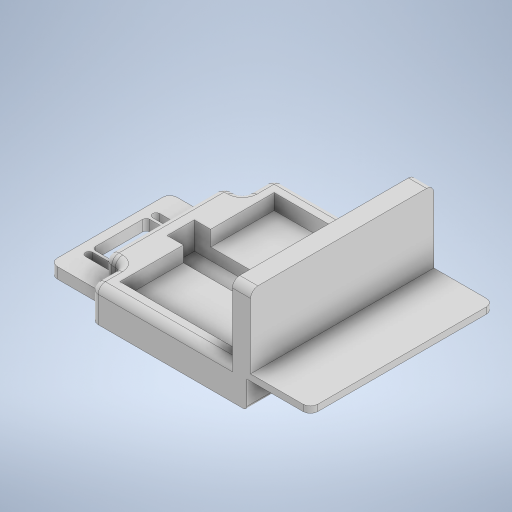
# Autodesk Inventor part: frame
Saved by Autodesk Inventor 2024 (Build 280153000, 153)
## iProperties
Created: 2024-11-23
Part Number: frame
Material: Generic
Document SubType Name: Modeling
Designer: tibs0
Density: 1 g/cm^3
Appearance: Default
Author: tibs0
Autodesk Inventor part; units mm, degrees
ref_plane "YZ Plane" through (0, 0, 0) normal (1, 0, 0) x (0, 1, 0)
ref_plane "XZ Plane" through (0, 0, 0) normal (0, 1, 0) x (-1, 0, 0)
ref_plane "XY Plane" through (0, 0, 0) normal (0, 0, 1) x (1, 0, 0)
sketch "Sketch1" plane through (0, 0, 0) normal (0, 1, 0) x (-1, 0, 0)
  line L0 (-35, 42.5) -> (35, 42.5)
  line L1 (35, 42.5) -> (35, -42.5)
  line L2 (35, -42.5) -> (-35, -42.5)
  line L3 (-35, -42.5) -> (-35, 42.5)
  line L4 (-35, 42.5) -> (35, -42.5) construction
  line L5 (35, 42.5) -> (-35, -42.5) construction
  line L6 (43, -50.5) -> (43, 50.5)
  line L7 (43, 50.5) -> (-43, 50.5)
  line L8 (-43, 50.5) -> (-43, -50.5)
  line L9 (-43, -50.5) -> (43, -50.5)
  line L10 (-43, -50.5) -> (-78, -50.5)
  line L11 (-78, -50.5) -> (-78, 50.5)
  line L12 (-78, 50.5) -> (-43, 50.5)
  line L13 (-43, 50.5) -> (-43, -50.5)
  point P0 (0, 0)
  point P1 (-43, 50.5)
  dimension "d0" = 70
  dimension "d1" = 85
  dimension "d2" = 8
  dimension "d13" = 35
  constraints: 28 end point, 6 parallel, 3 perpendicular, 2 horizontal, 2 midpoint, 3 other
  measures "d0" distance of L1.end L2.end
  measures "d1" distance of L0.end L1.end
  measures "d2" distance between parallel lines of L1 L6
  measures "d13" distance of L11.end L12.end
extrude "Extrusion1" add sketch "Sketch1" along normal blind 10 contours L0 L1 L2 L3
extrude "Extrusion2" add sketch "Sketch1" along normal blind 18.5
sketch "Sketch5" plane through (-43, 0, 50.5) normal (0, 0, 1) x (1, 0, 0)
  line L0 (0, 0) -> (121, 0) projected
  line L1 (121, 0) -> (121, 18.5) projected
  line L2 (0, 18.5) -> (121, 18.5) projected
  line L3 (0, 0) -> (0, 18.5) projected
  line L4 (78, 10) -> (78, 18.5) projected
  line L5 (121, 0) -> (86, 0)
  line L6 (86, 0) -> (86, 15)
  line L7 (86, 15) -> (121, 15)
  line L8 (121, 15) -> (121, 0)
  point P0 (43, 0)
  point P1 (86, 0)
  dimension "d14" = 35
  dimension "d15" = 15
  constraints: 8 end point, 2 parallel, 1 horizontal, 1 perpendicular
  measures "d14" distance of L6.end L7.end
  measures "d15" distance of L5.end L6.end
extrude "Extrusion5" cut sketch "Sketch5" against normal blind 101 contours L6 L7 L1 L0
sketch "Sketch6" plane through (0, 18.5, 0) normal (0, 1, 0) x (1, 0, 0)
  line L0 (-43, -50.5) -> (78, -50.5) projected
  line L1 (78, -50.5) -> (78, 50.5) projected
  line L2 (78, 50.5) -> (-43, 50.5) projected
  line L3 (-43, 50.5) -> (-43, -50.5) projected
  line L4 (35, -42.5) -> (-35, -42.5) projected
  line L5 (-35, -42.5) -> (-35, 42.5) projected
  line L6 (-35, 42.5) -> (35, 42.5) projected
  line L7 (35, 42.5) -> (35, -42.5) projected
  line L8 (35, 50.5) -> (45, 50.5)
  line L9 (45, 50.5) -> (45, -50.5)
  line L10 (45, -50.5) -> (35, -50.5)
  line L11 (35, -50.5) -> (35, 50.5)
  point P0 (0, 0)
  point P1 (35, -42.5)
  dimension "d18" = 10
  dimension "d21" = 0
  constraints: 8 end point, 2 parallel, 2 point on line, 1 horizontal, 1 perpendicular
  measures "d18" distance of L9.end L10.end
  measures "d21" distance between parallel lines of L7 L11
extrude "Extrusion6" add sketch "Sketch6" along normal blind 40 contours L11 L7 L2 L9 L0
sketch "Sketch8" plane through (-43, 18.5, 50.5) normal (0, 0, 1) x (1, 0, 0)
  line L0 (86, -3.5) -> (121, -3.5) projected
  line L1 (121, -3.5) -> (121, 0) projected
  line L2 (88, 0) -> (121, 0) projected
  line L3 (88, 0) -> (88, 40) projected
  line L4 (78, 40) -> (88, 40) projected
  line L5 (78, 0) -> (78, 40) projected
  line L6 (0, 0) -> (78, 0) projected
  line L7 (0, -18.5) -> (0, 0) projected
  line L8 (0, -18.5) -> (86, -18.5) projected
  line L9 (86, -18.5) -> (86, -3.5) projected
  line L10 (121, -3.5) -> (86, -3.5) projected
  line L11 (101.2519, -3.5) -> (101.2519, -33.5)
  line L12 (101.2519, -33.5) -> (-48.597, -33.5)
  line L13 (-48.597, -30.5) -> (-20.6061, -30.5)
  line L14 (-48.597, -27.5) -> (-20.6061, -27.5)
  point P0 (43, -18.5)
  dimension "d25" = 30
  dimension "d26" = 3
  dimension "d27" = 3
  constraints: 8 end point, 2 perpendicular, 1 horizontal, 1 parallel, 1 point on line
  measures "d25" distance of L11.start L11.end
  measures "d26" distance between parallel lines of L12 L13
  measures "d27" distance between parallel lines of L13 L14
sketch "Sketch9" plane through (-43, 0, -50.5) normal (-1, 0, 0) x (0, 0, 1)
  line L0 (0, 0) -> (101, 0) projected
  line L1 (101, 0) -> (101, 18.5) projected
  line L2 (0, 18.5) -> (101, 18.5) projected
  line L3 (0, 0) -> (0, 18.5) projected
  point P0 (50.5, 0)
extrude "Extrusion8" add sketch "Sketch9" along normal blind 40
sketch "Sketch10" plane through (0, 0, 0) normal (0, -1, 0) x (1, 0, 0)
  line L0 (43, -50.5) -> (43, 50.5) projected
  line L1 (-83, 50.5) -> (43, 50.5) projected
  line L2 (-83, -50.5) -> (-83, 50.5) projected
  line L3 (43, -50.5) -> (-83, -50.5) projected
  line L4 (-43, 50.5) -> (-43, -50.5)
  line L5 (43, -50.5) -> (-83, -50.5) projected
  point P0 (0, 0)
  point P1 (-43, -50.5)
  constraints: 2 end point, 1 perpendicular, 1 point on line
extrude "Extrusion9" add sketch "Sketch10" along normal blind 7 contours L3 L2 L1 L4
sketch "Sketch11" plane through (-83, 0, -50.5) normal (-1, 0, 0) x (0, 0, 1)
  line L0 (101, 18.5) -> (101, -7) projected
  line L1 (101, 18.5) -> (0, 18.5) projected
  line L2 (0, 18.5) -> (0, -7) projected
  line L3 (101, -7) -> (0, -7) projected
  line L4 (50.5, -7) -> (83.5, -7)
  line L5 (0, -7) -> (101, -7) projected
  line L6 (50.5, -7) -> (17.5, -7)
  line L7 (17.5, -1) -> (32, -1)
  line L8 (83.5, -1) -> (69, -1)
  line L9 (17.5, -7) -> (17.5, 18.5)
  line L10 (83.5, -7) -> (83.5, 18.5)
  line L11 (32, -1) -> (69, -1)
  line L12 (32, -1) -> (32, -7)
  line L13 (69, -1) -> (69, -7)
  point P0 (50.5, 0)
  dimension "d32" = 33
  dimension "d33" = 33
  dimension "d34" = 14.5
  dimension "d36" = 14.5
  dimension "d39" = 6
  dimension "d40" = 6
  constraints: 18 end point, 6 point on line, 4 perpendicular, 2 horizontal, 1 midpoint
  measures "d32" distance of L4.start L4.end
  measures "d33" distance of L4.start L6.end
  measures "d34" distance of L7.start L7.end
  measures "d36" distance of L8.start L8.end
  measures "d39" distance between parallel lines of L3 L7
  measures "d40" distance between parallel lines of L3 L8
extrude "Extrusion10" cut sketch "Sketch11" against normal blind 40 contours L0 L3 L10 L1 | L9 L3 L2 L1
extrude "Extrusion11" cut sketch "Sketch11" against normal blind 30 contours L10 L8 L11 L7 L9 L1
sketch "Sketch12" plane through (-83, -1, 33) normal (0, 1, 0) x (1, 0, 0)
  line L0 (0, 0) -> (0, 66) projected
  line L1 (30, 0) -> (0, 0) projected
  line L2 (30, 0) -> (30, 66) projected
  line L3 (0, 66) -> (30, 66) projected
  line L4 (5, 48) -> (30, 48)
  line L5 (30, 48) -> (30, 18)
  line L6 (30, 18) -> (5, 18)
  line L7 (5, 18) -> (5, 48)
  line L8 (5, 48) -> (30, 18) construction
  line L9 (30, 48) -> (5, 18) construction
  line L10 (5, 53.5) -> (30, 53.5)
  line L11 (30, 53.5) -> (30, 49.5)
  line L12 (30, 49.5) -> (5, 49.5)
  line L13 (5, 49.5) -> (5, 53.5)
  line L14 (5, 53.5) -> (30, 49.5) construction
  line L15 (30, 53.5) -> (5, 49.5) construction
  line L16 (5, 16.5) -> (30, 16.5)
  line L17 (30, 16.5) -> (30, 12.5)
  line L18 (30, 12.5) -> (5, 12.5)
  line L19 (5, 12.5) -> (5, 16.5)
  line L20 (5, 16.5) -> (30, 12.5) construction
  line L21 (30, 16.5) -> (5, 12.5) construction
  point P0 (83, 33)
  point P1 (0, 51.5)
  point P2 (0, 51.5)
  point P3 (0, 51.5)
  point P4 (0, 14.5)
  point P5 (0, 14.5)
  point P6 (0, 14.5)
  point P7 (17.5, 33)
  point P8 (30, 18)
  point P9 (17.5, 51.5)
  point P10 (17.5, 14.5)
  point P11 (30, 16.5)
  point P12 (30, 53.5)
  dimension "d43" = 25
  dimension "d44" = 0
  dimension "d47" = 30
  dimension "d48" = 18
  dimension "d49" = 4
  dimension "d50" = 4
  constraints: 36 end point, 6 midpoint, 6 parallel, 3 horizontal, 3 perpendicular, 2 point on line
  measures "d43" distance of L5.end L6.end
  measures "d44" distance between parallel lines of L2 L5
  measures "d47" distance of L4.end L5.end
  measures "d48" distance between parallel lines of L3 L4
  measures "d49" distance of L10.end L11.end
  measures "d50" distance of L16.end L17.end
extrude "Extrusion12" cut sketch "Sketch12" against normal blind 30 contours L6 L7 L4 L2
extrude "Extrusion13" cut sketch "Sketch12" against normal blind 30 contours L18 L19 L16 L2 | L2 L12 L13 L10
fillet "Fillet1" radius 2 6 edges at (-53, -4, -20.5) (-53, -4, 16.5) (-78, -4, -20.5) (-78, -4, -15) (-53, -4, -16.5) (-78, -4, -16.5)
fillet "Fillet2" radius 2 5 edges at (-53, -4, 20.5) (-53, -4, 15) (-78, -4, 15) (-78, -4, 20.5) (-78, -4, 16.5)
fillet "Fillet3" radius 4 9 edges at (-83, -4, 33) (-43, 9.25, 50.5) (-83, -4, -33) (78, 16.75, 50.5) (-4, 18.5, 50.5) (-53, 18.5, 0) (-43, 9.25, -50.5) (-4, 18.5, -50.5) (78, 16.75, -50.5)
fillet "Fillet4" radius 4 1 edges at (-43, -7, 0)
fillet "Fillet5" radius 4 2 edges at (40, 58.5, -50.5) (40, 58.5, 50.5)
sketch "Sketch15" plane through (-35, 10, -42.5) normal (1, 0, 0) x (0, 0, -1)
  line L0 (0, 0) -> (-85, 0) projected
  line L1 (-85, 8.5) -> (0, 8.5) projected
  line L2 (0, 0) -> (-85, 0) projected
  line L3 (0, 0) -> (0, 8.5) projected
  line L4 (-85, 8.5) -> (0, 8.5) projected
  line L5 (-85, 0) -> (-85, 8.5) projected
  line L6 (-50, 8.5) -> (-35, 8.5)
  line L7 (-35, 8.5) -> (-35, -6.5)
  line L8 (-35, -6.5) -> (-50, -6.5)
  line L9 (-50, -6.5) -> (-50, 8.5)
  point P0 (-42.5, -10)
  point P1 (-50, 8.5)
  point P2 (-50, 0)
  point P3 (-35, 0)
  dimension "d67" = 15
  dimension "d68" = 15
  dimension "d69" = 35
  constraints: 8 end point, 2 parallel, 1 horizontal, 1 perpendicular, 1 point on line
  measures "d67" distance of L7.end L8.end
  measures "d68" distance of L6.end L7.end
  measures "d69" distance between parallel lines of L3 L7
extrude "Extrusion14" cut sketch "Sketch15" along normal blind 78 and the other way blind 9 contours L7 L8 L9 L0 | L0 L9 L1 L7
fillet "Fillet6" radius 2 1 edges at (43, 0, 0)
fillet "Fillet7" radius 2 1 edges at (-53, -4, -15)
fillet "Fillet8" radius 4 2 edges at (-43, 9.25, -33) (-43, 9.25, 33)
fillet "Fillet9" radius 4 12 edges at (-51.8284, 17.3284, 33) (-48, 18.5, 33) (-44.1716, 18.5, 34.1716) (-43, 18.5, 41.75) (-41.8284, 17.3284, 49.3284) (-53, 6.75, 33) (-51.8284, 17.3284, -33) (-48, 18.5, -33) (-44.1716, 18.5, -34.1716) (-43, 18.5, -41.75) (-41.8284, 17.3284, -49.3284) (-53, 6.75, -33)
body "Solid1"
